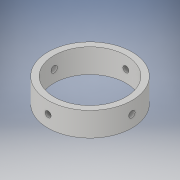
# Autodesk Inventor part: RounedInnerRing
Saved by Autodesk Inventor 2017 SP1 (Build 210196100, 196)
## iProperties
Created: 2016-07-31
Part Number: RounedInnerRing
Material: Generic
Document SubType Name: Modeling
Designer: steele
Density: 1 g/cm^3
Appearance: Default
Author: steele
Autodesk Inventor part; units mm, degrees
ref_plane "XZ Plane" through (0, 0, 0) normal (0, 1, 0) x (-1, 0, 0)
sketch "Sketch1" plane through (0, 0, 0) normal (0, 1, 0) x (-1, 0, 0)
  circle A0 centre (0, 0) radius 38.1
  circle A1 centre (0, 0) radius 44.45
  dimension "d0" = 76.2
  dimension "d1" = 88.9
  constraints: 2 centre point, 2 coincident
  measures "d0" diameter of A0
  measures "d1" diameter of A1
extrude "Extrusion1" add sketch "Sketch1" along normal mid plane 25.4
ref_plane "Work Plane1" through (0, 0, 44.45) normal (0, 0, 1) x (1, 0, 0)
sketch "Sketch2" plane through (0, 0, 44.45) normal (0, 0, 1) x (1, 0, 0)
  point P0 (0, 0)
  point P1 (0, 0)
  constraints: 1 coincident
hole "Hole1" at (0, 0, 44.45) direction (0, 0, -1) diameter 6.35 end through all
ref_plane "Work Plane2" through (44.45, 0, 0) normal (1, 0, 0) x (0, 1, 0)
sketch "Sketch3" plane through (44.45, 0, 0) normal (1, 0, 0) x (0, 1, 0)
  point P0 (0, 0)
  point P1 (0, 0)
  constraints: 1 coincident
hole "Hole2" at (44.45, 0, 0) direction (-1, 0, 0) diameter 6.7564 end through all clearance for "Flat Head Machine Screw (82)" size "1/4" standard "Ansi Unified Screw Threads"
equation "\"d0\" = cupDiam"
equation "\"d1\" = outerRingDism"
equation "\"d2\" = ringHeight"
equation "\"d5\" = ringAxelDiam"
equation "\"cupDiam\" = 76.2"
equation "\"ringThickness\" = 6.35"
equation "\"ringHeight\" = 25.4"
equation "\"ringAxelDiam\" = 6.35"
equation "\"outerRingDism\" = cupDiam + 2 * ringThickness"
equation "\"outerRingRadius\" = 0.5 * outerRingDism"
equation "\"d4\" = outerRingRadius"
equation "\"d12\" = outerRingRadius"
body "Solid1"
